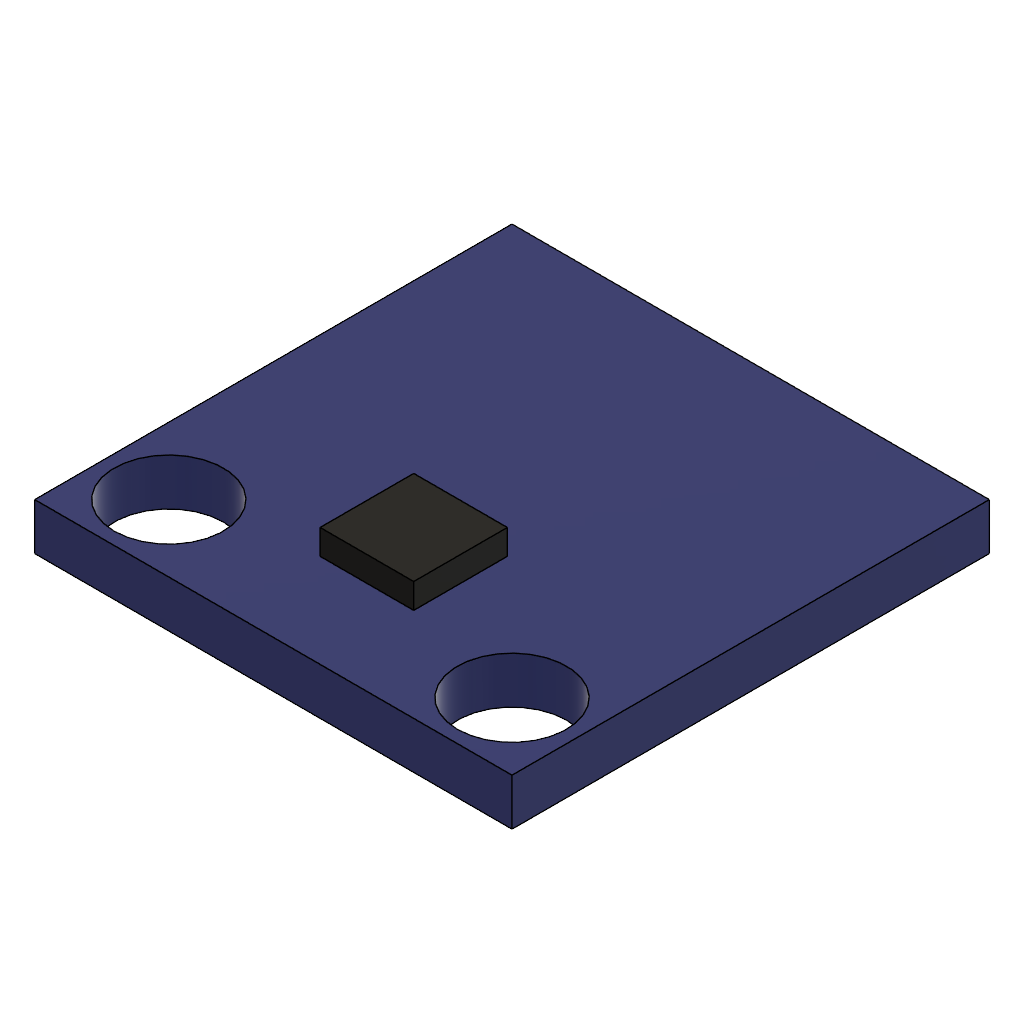
HTU21DBreakoutBoard (Autodesk Fusion 360 design; units mm, degrees)
part number: 2026-08-16-16-12-45-411
Autodesk Fusion 360 part; units mm, degrees
sketch "Sketch1" plane through (0, 0, 0) normal (0, 1, 0) x (1, 0, 0)
  line L0 (7.65, 7.65) -> (-7.65, 7.65)
  line L1 (-7.65, 7.65) -> (-7.65, -7.65)
  line L2 (-7.65, -7.65) -> (7.65, -7.65)
  line L3 (7.65, -7.65) -> (7.65, 7.65)
  line L4 (7.65, 7.65) -> (-7.65, -7.65) construction
  line L5 (-7.65, 7.65) -> (7.65, -7.65) construction
  dimension "d1" = 15.3
  dimension "d2" = 15.3
  constraint horizontal L0
  constraint perpendicular L0 L1
  constraint parallel L0 L2
  constraint parallel L1 L3
  constraint coincident L4 origin
  constraint coincident L5 origin
  measures "d1" distance of L1.end L2.end
  measures "d2" distance of L0.end L1.end
extrude "Extrude1" add sketch "Sketch1" along normal blind 1.5 makes body 1
hole "Hole1" at (-5.5, 1.5, 5.5) direction (0, -1, 0) diameter 3.5 depth 3.5 tip angle 118 bodies 1
hole "Hole2" at (5.5, 1.5, 5.5) direction (0, -1, 0) diameter 3.5 depth 3.5 tip angle 118 bodies 1
sketch "Sketch2" plane through (0, 1.5, 0) normal (0, 1, 0) x (-1, 0, 0)
  circle A0 centre (-5.5, 5.5) radius 1.75
  circle A1 centre (5.5, 5.5) radius 1.75
  line L0 (-7.65, 7.65) -> (-7.65, -7.65)
  line L1 (-7.65, -7.65) -> (7.65, -7.65)
  line L2 (7.65, -7.65) -> (7.65, 7.65)
  line L3 (7.65, 7.65) -> (-7.65, 7.65)
  line L4 (0, 7.65) -> (0, 4.65)
  line L5 (0, 4.65) -> (0, 3.15)
  line L6 (-1.5, 1.65) -> (1.5, 1.65)
  line L7 (1.5, 1.65) -> (1.5, 4.65)
  line L8 (1.5, 4.65) -> (-1.5, 4.65)
  line L9 (-1.5, 4.65) -> (-1.5, 1.65)
  line L10 (-1.5, 1.65) -> (1.5, 4.65) construction
  line L11 (1.5, 1.65) -> (-1.5, 4.65) construction
  point P0 (0, 3.15)
  dimension "d15" = 3
  dimension "d16" = 1.5
  dimension "d17" = 3
  dimension "d18" = 3
  constraint midpoint L3 L4.start
  constraint perpendicular L3 L4
  constraint parallel L4 L5
  constraint horizontal L6
  constraint perpendicular L6 L7
  constraint parallel L6 L8
  constraint parallel L7 L9
  constraint coincident L10 P0
  constraint coincident L11 P0
  constraint coincident P0 L5.end
  measures "d15" distance of L4.start L4.end
  measures "d16" distance of L4.end P0
  measures "d17" distance of L7.end L8.end
  measures "d18" distance of L6.end L7.end
extrude "Extrude2" add sketch "Sketch2" along normal blind 0.8 separate body contours L6 L7 L8 L9 makes body 2
